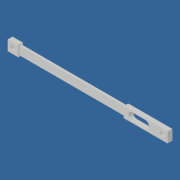
# Autodesk Inventor part: KON_Nietmaschine_Hebel
Saved by Autodesk Inventor 2019 (Build 230136000, 136)
## iProperties
Created: 2021-12-12
Part Number: KON_Nietmaschine_Hebel
Material: Generisch
Document SubType Name: Modeling
Designer: Jonas Nebl
Density: 1 g/cm^3
Appearance: Vorgabe
Mass: 302.09 g
Surface Area: 750.704 cm^2
Volume: 302.09 cm^3
Author: Jonas Nebl
Autodesk Inventor part; units mm, degrees
ref_plane "YZ Plane" through (0, 0, 0) normal (1, 0, 0) x (0, 1, 0)
ref_plane "XZ Plane" through (0, 0, 0) normal (0, 1, 0) x (-1, 0, 0)
ref_plane "XY Plane" through (0, 0, 0) normal (0, 0, 1) x (1, 0, 0)
sketch "Skizze1" plane through (0, 0, 0) normal (0, 0, 1) x (1, 0, 0)
  line L0 (-350, 0) -> (-350, -22.5)
  line L1 (-350, -22.5) -> (-305, -22.5)
  line L2 (-305, -22.5) -> (-305, -17.5)
  line L3 (-305, -17.5) -> (158.3583, -17.5)
  line L4 (158.3583, -22.5) -> (350, -22.5)
  line L5 (350, 0) -> (350, -22.5)
  line L6 (158.3583, -17.5) -> (158.3583, -22.5)
  arc A0 (-337.5, 0) -> (-317.5, 0) centre (-327.5, 0) ccw
  line L7 (-490, 0) -> (490, 0) projected
  line L8 (-350, 0) -> (-337.5, 0)
  arc A1 (317.5, 0) -> (337.5, 0) centre (327.5, 0) ccw
  line L9 (337.5, 0) -> (350, 0)
  arc A2 (178.207, 0) -> (196.1598, -17.9528) centre (196.1598, 0) ccw
  arc A3 (252.2039, -17.9528) -> (270.1567, 0) centre (252.2039, 0) ccw
  line L10 (196.1598, -17.9528) -> (252.2039, -17.9528)
  line L11 (-317.5, 0) -> (178.207, 0)
  line L12 (270.1567, 0) -> (317.5, 0)
  point P0 (0, 0)
  dimension "d0" = 700
  dimension "d1" = 17.5
  dimension "d2" = 10
  dimension "d3" = 10
  dimension "d4" = 5
  dimension "d5" = 5
  dimension "d6" = 45
  dimension "d7" = 22.5
  dimension "d8" = 350
  dimension "d9" = 22.5
  constraints: 24 end point, 8 point on circle, 7 horizontal, 4 centre point, 4 vertical, 2 tangent, 1 point on line, 12 other
  measures "d0" distance between parallel lines of L5 L0
  measures "d1" distance of the line from the sketch origin of L3
  measures "d2" radius of A0
  measures "d3" radius of A1
  measures "d4" distance of L1.end L2.end
  measures "d5" distance of L3.end L4.start
  measures "d6" distance of L0.end L1.end
  measures "d7" distance from line of L0 A0.centre
  measures "d8" distance from line of point (0, 0) L0
  measures "d9" distance from line of L5 A1.centre
extrude "Extrusion1" add sketch "Skizze1" along normal mid plane 20 contours L7 A0 A2 L10 A3 A1 L5 L4 L6 L3 L2 L1 L0
mirror "Spiegeln1" about plane through (0, 0, 0) normal (0, 1, 0)
sketch "Skizze2" plane through (0, 0, 0) normal (0, 1, 0) x (-1, 0, 0)
  line L0 (-158.3583, -10) -> (-158.3583, 10) projected
  line L1 (305, 10) -> (-158.3583, 10) projected
  line L2 (305, -10) -> (305, 10) projected
  line L3 (-158.3583, -10) -> (305, -10) projected
  line L4 (305, -10) -> (305, 10) projected
  line L5 (-158.3583, -10) -> (-158.3583, 10) projected
  line L6 (305, -10) -> (-158.3583, -10)
  line L7 (-158.3583, -10) -> (-158.3583, -5)
  line L8 (-158.3583, -5) -> (305, -5)
  line L9 (305, -5) -> (305, -10)
  line L10 (305, 10) -> (-158.3583, 10)
  line L11 (-158.3583, 10) -> (-158.3583, 5)
  line L12 (-158.3583, 5) -> (305, 5)
  line L13 (305, 5) -> (305, 10)
  line L14 (397.6717, 0) -> (-251.03, 0) projected
  point P0 (0, 0)
  dimension "d12" = 10
  constraints: 16 end point, 4 parallel, 2 horizontal, 2 perpendicular, 2 point on line, 1 other
  measures "d12" distance between parallel lines of L12 L8
extrude "Extrusion2" cut sketch "Skizze2" along normal through all both and the other way through all contours L0 L8 L2 L3 | L0 L1 L2 L12
equation "\"d0\" = lges"
equation "\"d1\" = 0.5 * h_Hebelprofil"
equation "\"d2\" = r_Lager"
equation "\"d3\" = r_Lager"
equation "\"d8\" = 0.5 * lges"
equation "\"d12\" = b_Hebelprofil"
equation "\"lges\" = 700"
equation "\"h_Hebelprofil\" = 35"
equation "\"b_Hebelprofil\" = 10"
equation "\"r_Lager\" = 10"
